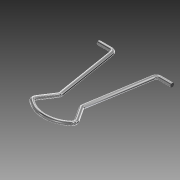
# Autodesk Inventor part: BINDER CLIP ARM
Saved by Autodesk Inventor 2013 (Build 170138000, 138)
## iProperties
Created: 2014-06-22
Part Number: BINDER CLIP ARM
Material: Generic
Document SubType Name: Modeling
Designer: employee
Density: 1 g/cm^3
Author: employee
Autodesk Inventor part; units mm, degrees
ref_plane "YZ Plane" through (0, 0, 0) normal (1, 0, 0) x (0, 1, 0)
ref_plane "XZ Plane" through (0, 0, 0) normal (0, 1, 0) x (-1, 0, 0)
ref_plane "XY Plane" through (0, 0, 0) normal (0, 0, 1) x (1, 0, 0)
sketch "Sketch1" plane through (0, 0, 0) normal (0, 0, 1) x (1, 0, 0)
  line L0 (0, 0) -> (-17.2455, 0) construction
  arc A0 (0, 0) -> (7.9502, 2.8394) centre (0, 12.55) ccw
  arc A1 (7.9502, 2.8394) -> (8.2547, 4.8221) centre (7, 4) ccw
  line L1 (8.2547, 4.8221) -> (4.7453, 10.1779)
  arc A2 (4.5196, 11.2417) -> (4.7453, 10.1779) centre (6, 11) ccw
  line L2 (4.5196, 11.2417) -> (8.5196, 35.7417)
  arc A3 (10, 37) -> (8.5196, 35.7417) centre (10, 35.5) ccw
  line L3 (10, 37) -> (15, 37)
  dimension "d0" = 7
  dimension "d1" = 6
  dimension "d2" = 10
  dimension "d3" = 1.5
  dimension "d4" = 37
  dimension "d5" = 11
  dimension "d6" = 4
  dimension "d10" = 5
  constraints: 8 end point, 8 point on circle, 7 tangent, 4 centre point, 2 equal radius, 1 horizontal, 1 parallel
  measures "d0" horizontal distance of A1.centre L0.start
  measures "d1" horizontal distance of A2.centre L0.start
  measures "d2" horizontal distance of A3.centre L0.start
  measures "d3" radius of A2
  measures "d4" distance from line of L3 L0.start
  measures "d5" vertical distance of A2.centre L0.start
  measures "d6" vertical distance of A1.centre L0.start
  measures "d10" distance of L3.start L3.end
sketch "Sketch2" plane through (0, 0, 0) normal (1, 0, 0) x (0, 1, 0)
  circle A0 centre (0, 0) radius 0.75
  dimension "d7" = 1.5
  constraints: 1 centre point, 1 coincident
  measures "d7" diameter of A0
sweep "Sweep1" add profiles "Sketch2" path "Sketch1"
mirror "Mirror1" about plane through (0, 0, 0) normal (-1, 0, 0) of "Sweep1"
body "Solid1"
